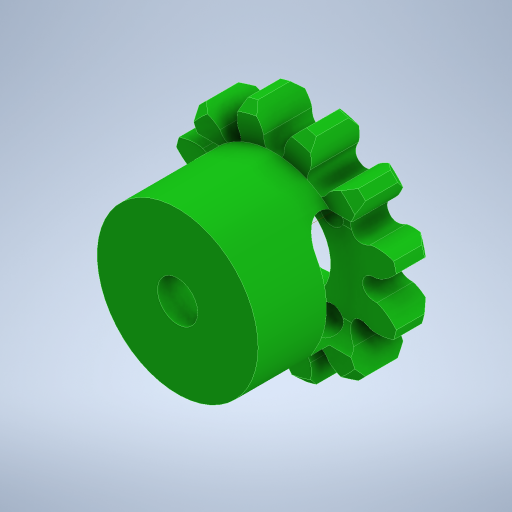
# Autodesk Inventor part: шестерня12_туу
Saved by Autodesk Inventor 2024 (Build 280153000, 153)
## iProperties
Created: 2025-10-14
Part Number: шестерня12_туу
Material: Generic
Document SubType Name: Modeling
Designer: DELL
Density: 1 g/cm^3
Appearance: Темно-зеленый
Author: DELL
Autodesk Inventor part; units mm, degrees
ref_plane "YZ Plane" through (0, 0, 0) normal (1, 0, 0) x (0, 1, 0)
ref_plane "XZ Plane" through (0, 0, 0) normal (0, 1, 0) x (-1, 0, 0)
sketch "Sketch1" plane through (0, 0, 0) normal (0, 0, 1) x (1, 0, 0)
  spline S0 degree 3 poles (-3.0087, 13.6604) (-2.9154, 13.5764) (-2.7289, 13.4085) (-2.4652, 13.1397) (-2.215, 12.8584) (-1.9815, 12.563) (-1.7672, 12.2533) (-1.608, 11.9827) (-1.4953, 11.7584) (-1.42, 11.586) (-1.3534, 11.4097) (-1.324, 11.2876) (-1.3093, 11.2266) knots 0 0 0 0 0.037634 0.075268 0.112902 0.150535 0.188166 0.225794 0.244611 0.263428 0.282243 0.30105 0.30105 0.30105 0.30105
  spline S1 degree 3 poles (-1.3093, 11.2266) (-1.3081, 11.1237) (-1.3062, 10.9693) (-1.2835, 10.7645) (-1.2555, 10.6127) (-1.2209, 10.4621) (-1.1712, 10.3158) (-1.1128, 10.1727) (-1.0388, 10.037) (-0.951, 9.9097) (-0.8483, 9.794) (-0.7312, 9.6929) (-0.6003, 9.6102) (-0.4585, 9.5481) (-0.3086, 9.5088) (-0.1543, 9.4971) (0, 9.5015) (0.1543, 9.4971) (0.3086, 9.5088) (0.4585, 9.5481) (0.6003, 9.6102) (0.7312, 9.6929) (0.8483, 9.794) (0.951, 9.9097) (1.0388, 10.037) (1.1128, 10.1727) (1.1712, 10.3158) (1.2209, 10.4621) (1.2555, 10.6127) (1.2835, 10.7645) (1.3062, 10.9693) (1.3081, 11.1237) (1.3093, 11.2266) knots 0 0 0 0 0.03086 0.046295 0.061729 0.077164 0.092597 0.10803 0.123465 0.138895 0.154322 0.169746 0.185167 0.200585 0.215997 0.231413 0.246848 0.262284 0.2777 0.293112 0.30853 0.323951 0.339375 0.354802 0.370232 0.385667 0.4011 0.416533 0.431968 0.447402 0.462836 0.493697 0.493697 0.493697 0.493697
  spline S2 degree 3 poles (1.3093, 11.2266) (1.324, 11.2876) (1.3534, 11.4097) (1.42, 11.586) (1.4953, 11.7584) (1.608, 11.9827) (1.7672, 12.2533) (1.9815, 12.563) (2.215, 12.8584) (2.4652, 13.1397) (2.7289, 13.4085) (2.9154, 13.5764) (3.0087, 13.6604) knots 0 0 0 0 0.018807 0.037622 0.056439 0.075256 0.112884 0.150515 0.188148 0.225782 0.263416 0.30105 0.30105 0.30105 0.30105
  circle A0 centre (0, 0) radius 9.5 construction
  circle A1 centre (0, 0) radius 11.2763 construction
  circle A2 centre (0, 0) radius 12 construction
  circle A3 centre (0, 0) radius 13.9878
  point P0 (-2.7316, 13.4057)
  point P1 (-2.4675, 13.1376)
  point P2 (-2.2178, 12.856)
  point P3 (-1.9847, 12.5606)
  point P4 (-1.7711, 12.2508)
  point P5 (-1.5811, 11.926)
  point P6 (-1.4968, 11.7577)
  point P7 (-1.4215, 11.5853)
  point P8 (-1.3572, 11.4085)
  point P9 (-1.2988, 10.9182)
  point P10 (-1.2817, 10.7648)
  point P11 (-1.2544, 10.6129)
  point P12 (-1.2184, 10.4628)
  point P13 (-1.1698, 10.3163)
  point P14 (-1.1102, 10.1739)
  point P15 (-1.0365, 10.0384)
  point P16 (-0.9485, 9.9116)
  point P17 (-0.8459, 9.7964)
  point P18 (-0.7288, 9.6959)
  point P19 (-0.5984, 9.6136)
  point P20 (-0.4571, 9.5519)
  point P21 (-0.3079, 9.5134)
  point P22 (-0.1544, 9.4998)
  point P23 (0, 9.5)
  point P24 (0.1544, 9.4998)
  point P25 (0.3079, 9.5134)
  point P26 (0.4571, 9.5519)
  point P27 (0.5984, 9.6136)
  point P28 (0.7288, 9.6959)
  point P29 (0.8459, 9.7964)
  point P30 (0.9485, 9.9116)
  point P31 (1.0365, 10.0384)
  point P32 (1.1102, 10.1739)
  point P33 (1.1698, 10.3163)
  point P34 (1.2184, 10.4628)
  point P35 (1.2544, 10.6129)
  point P36 (1.2817, 10.7648)
  point P37 (1.2988, 10.9182)
  point P38 (1.3572, 11.4085)
  point P39 (1.4215, 11.5853)
  point P40 (1.4968, 11.7577)
  point P41 (1.5811, 11.926)
  point P42 (1.7711, 12.2508)
  point P43 (1.9847, 12.5606)
  point P44 (2.2178, 12.856)
  point P45 (2.4675, 13.1376)
  point P46 (2.7316, 13.4057)
  constraints: 4 centre point, 2 point on circle, 109 other
extrude "Выдавливание1" add sketch "Sketch1" against normal blind 6
extrude "Выдавливание2" cut sketch "Sketch1" against normal blind 10 contours A3 S2 S1 S0 picked at (-0.374, 12.578)
chamfer "Фаска1" distance 1 angle 45 2 edges at (0, -13.9878, 0) (0, -13.9878, -6)
pattern_circular "Круговой массив2" count 12 over 360 about axis through (0, 0, 0) along (0, 0, -1) of "Выдавливание2"
sketch "Эскиз2" plane through (0, 0, 0) normal (0, 0, 1) x (1, 0, 0)
  circle A0 centre (0, 0) radius 10
  dimension "d13" = 20
  constraints: 1 centre point, 1 coincident
  measures "d13" diameter of A0
extrude "Выдавливание3" add sketch "Эскиз2" along normal blind 12
sketch "Эскиз8" plane through (0, 0, -6) normal (0, 0, -1) x (-1, 0, 0)
  circle A0 centre (0, 0) radius 5.5
  dimension "d43" = 11
  constraints: 1 centre point, 1 coincident
  measures "d43" diameter of A0
extrude "Выдавливание9" cut sketch "Эскиз8" against normal blind 12
sketch "Эскиз9" plane through (0, 0, 6) normal (0, 0, -1) x (-1, 0, 0)
  circle A0 centre (0, 0) radius 2.5
  dimension "d46" = 5
  constraints: 1 centre point, 1 coincident
  measures "d46" diameter of A0
extrude "Выдавливание10" cut sketch "Эскиз9" against normal blind 10
sketch "Эскиз10" plane through (0, 0, -6) normal (0, 0, -1) x (-1, 0, 0)
  circle A0 centre (0, 0) radius 8 construction
  arc A1 (10.3259, 9.4358) -> (9.4358, 10.3259) centre (0, 0) ccw construction
  arc A2 (-10.3259, -9.4358) -> (-9.4358, -10.3259) centre (0, 0) ccw construction
  arc A3 (9.4358, -10.3259) -> (10.3259, -9.4358) centre (0, 0) ccw construction
  arc A4 (-9.4358, 10.3259) -> (-10.3259, 9.4358) centre (0, 0) ccw construction
  line L0 (9.8908, 9.8908) -> (-9.8908, -9.8908) construction
  line L1 (9.8908, -9.8908) -> (-9.8908, 9.8908) construction
  circle A5 centre (-5.6569, 5.6569) radius 1.5
  circle A6 centre (-5.6569, -5.6569) radius 1.5
  circle A7 centre (5.6569, -5.6569) radius 1.5
  circle A8 centre (5.6569, 5.6569) radius 1.5
  dimension "d49" = 16
  dimension "d50" = 3
  dimension "d51" = 3
  dimension "d52" = 3
  dimension "d53" = 3
  constraints: 8 point on circle, 5 centre point, 4 end point, 4 point on line, 1 coincident
  measures "d49" diameter of A0
  measures "d50" diameter of A5
  measures "d51" diameter of A6
  measures "d52" diameter of A7
  measures "d53" diameter of A8
extrude "Выдавливание11" cut sketch "Эскиз10" against normal blind 10
ref_plane "РабПлоскость2" through (0, 0, -6) normal (1, 0, 0) x (0, 0, 1)
ref_plane "РабПлоскость1" through (5.6569, 5.6569, -6) normal (0.7071, -0.7071, 0) x (0, 0, 1)
sketch "Эскиз12" plane through (0, 0, -6) normal (1, 0, 0) x (0, 0, 1)
  line L0 (18, -10) -> (18, 10) construction
  line L1 (7, 5) -> (7, -5) construction
  line L2 (4.5, 5) -> (4.5, -5)
  line L3 (9.5, -5) -> (9.5, 5)
  arc A0 (9.5, 5) -> (4.5, 5) centre (7, 5) ccw
  arc A1 (4.5, -5) -> (9.5, -5) centre (7, -5) ccw
  line L4 (0, -5.5) -> (0, 5.5) projected
  point P0 (7, 0)
  dimension "d59" = 5
  dimension "d60" = 5
  dimension "d64" = 4.5
  constraints: 8 end point, 4 point on circle, 4 tangent, 2 centre point, 1 midpoint, 1 parallel, 1 vertical
  measures "d59" distance of point (7, 0) L1.end
  measures "d60" diameter of A1
  measures "d64" distance between parallel lines of L4 L2
extrude "Выдавливание12" cut sketch "Эскиз12" along normal mid plane 30
equation "\"Модуль\" = 2"
equation "\"Угол_зацепления\" = 20deg"
equation "\"Зазор_профиля_зуба\" = 0.25"
equation "\"Радиус_закругления_зуба\" = 0.35"
equation "\"Диаметр_головки\" = 27.97554"
equation "\"Диаметр_впадин\" = 19"
equation "\"Основной_диаметр\" = 22.55262"
equation "\"Средний_диаметр\" = 24"
equation "\"Коэффициент_смещения\" = 0"
equation "\"Изменение_высоты_головки_зуба\" = 0.006115"
equation "\"Окружной_шаг\" = 6.283185"
equation "\"Общий_сдвиг_инструмента\" = 0"
equation "\"Внутренний\" = 0"
